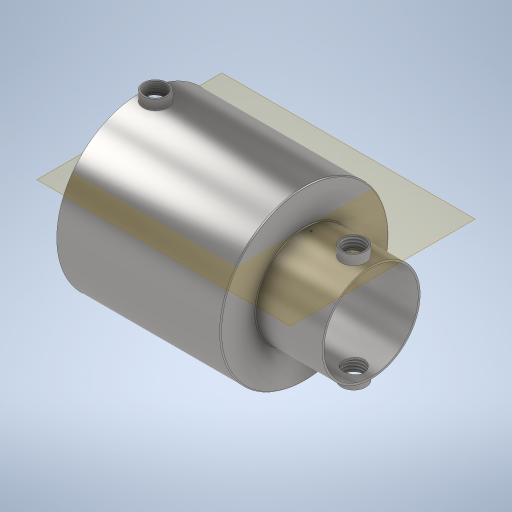
# Autodesk Inventor part: new outer wall
Saved by Autodesk Inventor 2023 (Build 270158000, 158)
## iProperties
Created: 2022-07-21
Part Number: new outer wall
Material: Stainless Steel
Document SubType Name: Modeling
Designer: station
Density: 8 g/cm^3
Appearance: Semi-Polished
Mass: 2032.08 g
Surface Area: 2551.28 cm^2
Volume: 254.01 cm^3
Author: station
Autodesk Inventor part; units mm, degrees
ref_plane "YZ Plane" through (0, 0, 0) normal (1, 0, 0) x (0, 1, 0)
ref_plane "XY Plane" through (0, 0, 0) normal (0, 0, 1) x (1, 0, 0)
sketch "Sketch1" plane through (0, 0, 0) normal (0, 0, 1) x (1, 0, 0)
  arc A0 (180.1312, 21.4516) -> (182.1847, 21.7676) centre (180.1312, 28.2803) ccw
  arc A1 (166.724, 25.044) -> (180.1312, 21.4516) centre (180.1312, 48.266) ccw
  line L0 (123.3912, 50.0622) -> (166.724, 25.044)
  arc A2 (123.3912, 50.0622) -> (30.0219, 75.0805) centre (30.0219, -111.6581) ccw
  line L1 (0, 75.0805) -> (30.0219, 75.0805)
  line L2 (0, 3.5755) -> (0, 203.5755) construction
  line L3 (0, 3.5755) -> (319.1694, 3.5755)
  line L4 (0, 77.0805) -> (30.0219, 77.0805)
  arc A3 (124.3912, 51.7943) -> (30.0219, 77.0805) centre (30.0219, -111.6581) ccw
  line L5 (124.3912, 51.7943) -> (167.724, 26.7761)
  arc A4 (167.724, 26.7761) -> (180.1312, 23.4516) centre (180.1312, 48.266) ccw
  arc A5 (180.1312, 23.4516) -> (181.5842, 23.6753) centre (180.1312, 28.2803) ccw
  line L6 (182.1847, 21.7676) -> (237.115, 39.0871)
  line L7 (236.5136, 40.9945) -> (181.5833, 23.6751)
  arc A6 (180.1312, 23.4516) -> (181.5833, 23.6751) centre (180.1312, 28.2803) ccw
  line L8 (236.5136, 40.9945) -> (237.115, 39.0871)
  line L9 (0, 88.1805) -> (30.0219, 88.1805)
  line L10 (166.724, 25.044) -> (166.724, -4.6444)
  line L11 (30.0219, 88.1805) -> (165.724, 88.1805)
  line L12 (237.115, 39.0871) -> (233.0254, 52.0576)
  line L13 (236.5136, 40.9945) -> (233.0254, 52.0576)
  line L14 (233.0254, 52.0576) -> (144.4694, 24.136)
  line L15 (233.0254, 52.0576) -> (237.115, 52.0576)
  line L16 (233.0254, 52.0576) -> (167.724, 52.0576)
  line L17 (167.724, 90.1805) -> (30.0219, 90.1805)
  line L18 (30.0219, 90.1805) -> (0, 90.1805)
  line L19 (233.0254, 54.0576) -> (169.724, 54.0576)
  line L20 (168.724, 25.044) -> (168.724, 31.7835)
  line L21 (168.724, 55.0576) -> (168.724, 89.1805)
  line L22 (166.724, 25.044) -> (166.724, 31.1529)
  line L23 (166.724, 53.0576) -> (166.724, 87.1805)
  arc A7 (166.724, 87.1805) -> (165.724, 88.1805) centre (165.724, 87.1805) ccw
  arc A8 (168.724, 89.1805) -> (167.724, 90.1805) centre (167.724, 89.1805) ccw
  arc A9 (168.724, 55.0576) -> (169.724, 54.0576) centre (169.724, 55.0576) ccw
  arc A10 (166.724, 53.0576) -> (167.724, 52.0576) centre (167.724, 53.0576) ccw
  line L24 (0, 88.1805) -> (0, 90.1805)
  line L25 (237.115, 52.0576) -> (237.115, 54.0576)
  line L26 (233.0254, 54.0576) -> (237.115, 54.0576)
  dimension "d48" = 200
  dimension "d49" = 30.0219
  dimension "d50" = 186.7386
  dimension "d51" = 0
  dimension "d52" = 0
  dimension "d53" = 0
  dimension "d54" = 71.505
  dimension "d55" = 2
  dimension "d56" = 2
  dimension "d57" = 2
  dimension "d58" = 2
  dimension "d59" = 2
  dimension "d60" = 17.5
  dimension "d61" = 54.9303
  dimension "d62" = 2
  dimension "d63" = 11.1
  dimension "d66" = 11.6
  dimension "d67" = 17.5
  dimension "d68" = 2
  dimension "d69" = 2
  dimension "d70" = 1
  dimension "d71" = 1
  dimension "d72" = 1
  dimension "d73" = 1
  constraints: 54 end point, 22 point on circle, 11 centre point, 9 tangent, 4 horizontal, 4 parallel, 4 vertical, 2 point on line, 1 collinear, 1 perpendicular, 2 other
  measures "d48" distance of L2.start L2.end
  measures "d49" distance of L1.start L1.end
  measures "d50" radius of A2
  measures "d51" distance from line of L1.start L2
  measures "d52" distance of A2.end L1.end
  measures "d53" distance of L0.start A2.start
  measures "d54" distance between parallel lines of L3 L1
  measures "d55" distance between parallel lines of L1 L4
  measures "d56" radial gap between concentric circles of A2 A3
  measures "d57" distance between parallel lines of L0 L5
  measures "d58" radial gap between concentric circles of A1 A4
  measures "d59" radial gap between concentric circles of A0 A5
  measures "d60" angle of L3 L6
  measures "d61" horizontal distance of L6.start L6.end
  measures "d62" distance between parallel lines of L6 L7
  measures "d63" distance between parallel lines of L4 L9
  measures "d66" distance of L12.end L7.start
  measures "d67" angle of L3 L14
  measures "d68" distance between parallel lines of L11 L17
  measures "d69" distance between parallel lines of L16 L19
  measures "d70" radius of A7
  measures "d71" radius of A8
  measures "d72" radius of A9
  measures "d73" radius of A10
revolve "Revolution3" add sketch "Sketch1" angle 360 about axis through (0, 3.5755, 0) along (1, 0, 0) contours L16 A10 L23 A7 L11 L9 L24 L18 L17 A8 L21 A9 L19 L26 L25 L15
sketch "Sketch5" plane through (0, 0, 0) normal (0, 0, 1) x (1, 0, 0)
  point P0 (0, 0)
ref_plane "Work Plane3" through (0, 90.18, 0) normal (0, 1, 0) x (-1, 0, 0)
sketch "Sketch7" plane through (0, 90.18, 0) normal (0, 1, 0) x (-1, 0, 0)
  circle A0 centre (-15, 0) radius 12.5
  circle A1 centre (-15, 0) radius 10.668
  line L0 (-167.724, 86.605) -> (-167.724, -86.605) projected
  point P0 (0, 0)
  dimension "d89" = 25
  dimension "d90" = 21.336
  dimension "d91" = 15
  dimension "d95" = 86.605
  constraints: 2 centre point, 1 coincident
  measures "d89" diameter of A0
  measures "d90" diameter of A1
  measures "d91" distance of A0.centre point (0, 0)
  measures "d95" vertical distance of L0.end A0.centre
extrude "Extrusion4" add sketch "Sketch7" along normal blind 10
ref_plane "Work Plane4" through (0, 3.575, 0) normal (0, 1, 0) x (-1, 0, 0)
mirror "Mirror1" about plane through (0, 3.575, 0) normal (0, 1, 0) of "Extrusion4"
ref_plane "Work Plane5" through (0, 54.057, 0) normal (0, 1, 0) x (-1, 0, 0)
sketch "Sketch8" plane through (0, 54.057, 0) normal (0, 1, 0) x (-1, 0, 0)
  circle A0 centre (-219.115, 0) radius 10.668
  circle A1 centre (-219.115, 0) radius 12.5
  line L0 (-237.115, 50.4822) -> (-237.115, -50.4822) projected
  point P0 (0, 0)
  dimension "d101" = 21.336
  dimension "d102" = 25
  dimension "d103" = 18
  dimension "d104" = 50.4821
  constraints: 2 centre point, 1 coincident
  measures "d101" diameter of A0
  measures "d102" diameter of A1
  measures "d103" distance from line of A0.centre L0
  measures "d104" vertical distance of L0.end A0.centre
extrude "Extrusion5" add sketch "Sketch8" along normal blind 10 separate body
mirror "Mirror2" about plane through (0, 3.575, 0) normal (0, 1, 0) of "Extrusion5" bodies 1
hole "Hole1" at (15, 90.18, 0) direction (0, -1, 0) diameter 21.336 end through all bodies 1
hole "Hole2" at (219.115, 54.057, 0) direction (0, -1, 0) diameter 21.336 end through all bodies 1
thread "Thread6" size "M15x1.5" class "6H" standard "ANSI Metric M Profile" full length
thread "Thread7" size "M15x1.5" class "6H" standard "ANSI Metric M Profile" full length
thread "Thread8" size "M22x3" class "6H" standard "ANSI Metric M Profile" full length
thread "Thread9" size "M22x3" class "6H" standard "ANSI Metric M Profile" full length
sketch "Sketch9" plane through (0, 54.057, 0) normal (0, 1, 0) x (-1, 0, 0)
  line L0 (11.8543, 0) -> (-175.1457, 0)
  circle A0 centre (-175.1457, 0) radius 1
  point P0 (0, 0)
  dimension "d129" = 187
  dimension "d130" = 2
  constraints: 2 end point, 1 centre point, 1 coincident, 1 horizontal
  measures "d129" distance of L0.start L0.end
  measures "d130" diameter of A0
hole "Hole3" at (175.1457, 54.057, 0) direction (0, -1, 0) diameter 2 depth 10 tip angle 118 bodies 1
thread "Thread10" size "M2x0.4" class "6H" standard "ANSI Metric M Profile" length 3
body "Solid3"
body "Solid4"
